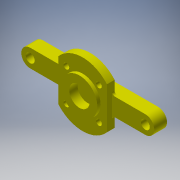
# Autodesk Inventor part: Coperchio inferiore
Saved by Autodesk Inventor 2016 (Build 200138000, 138)
## iProperties
Created: 2016-12-01
Part Number: Coperchio inferiore
Material: Generic
Document SubType Name: Modeling
Designer: Muhammad
Density: 1 g/cm^3
Appearance: Default
Author: Muhammad
Autodesk Inventor part; units mm, degrees
ref_plane "YZ Plane" through (0, 0, 0) normal (1, 0, 0) x (0, 1, 0)
ref_plane "XY Plane" through (0, 0, 0) normal (0, 0, 1) x (1, 0, 0)
sketch "Sketch1" plane through (0, 0, 0) normal (0, 1, 0) x (-1, 0, 0)
  line L0 (0, 0) -> (45, 0) construction
  line L1 (0, 0) -> (52, 0)
  line L2 (0, 0) -> (-45, 0)
  line L3 (-45, 0) -> (45, 0) construction
  line L4 (-45, -7) -> (45, -7)
  line L5 (45, 7) -> (-45, 7)
  arc A0 (-45, 7) -> (-45, -7) centre (-45, 0) ccw
  arc A1 (45, -7) -> (45, 7) centre (45, 0) ccw
  circle A2 centre (45, 0) radius 3.5
  circle A3 centre (-45, 0) radius 3.5
  dimension "d0" = 45
  dimension "d1" = 52
  dimension "d2" = 45
  dimension "d3" = 7
  constraints: 14 end point, 4 centre point, 4 point on circle, 4 tangent, 3 horizontal, 2 coincident, 1 collinear, 1 midpoint, 1 parallel
  measures "d0" distance of L0.start L0.end
  measures "d1" distance of L0.start L1.end
  measures "d2" distance of L0.start L2.end
  measures "d3" diameter of A2
extrude "Extrusion1" add sketch "Sketch1" along normal blind 10
ref_plane "Work Plane1" through (0, 2, 0) normal (0, 1, 0) x (-1, 0, 0)
sketch "Sketch2" plane through (0, 2, 0) normal (0, 1, 0) x (-1, 0, 0)
  line L0 (0, 0) -> (19, 0)
  line L1 (19, 0) -> (19, -16.2481)
  line L2 (19, 0) -> (19, 16.2481)
  line L3 (0, 0) -> (-19, 0)
  line L4 (-19, 0) -> (-19, -16.2481)
  line L5 (-19, 0) -> (-19, 16.2481)
  arc A0 (-19, -16.2481) -> (19, -16.2481) centre (0, 0) ccw
  arc A1 (19, 16.2481) -> (-19, 16.2481) centre (0, 0) ccw
  dimension "d8" = 19
  dimension "d10" = 19
  constraints: 12 end point, 4 point on circle, 2 centre point, 2 coincident, 2 horizontal, 2 point on line, 1 perpendicular, 1 vertical
  measures "d8" distance of L0.start L0.end
  measures "d10" distance of L3.start L3.end
extrude "Extrusion2" add sketch "Sketch2" against normal blind 6
fillet "Fillet1" radius 2 4 edges at (-19, 1, -7) (-19, 1, 7) (19, 1, -7) (19, 1, 7)
sketch "Sketch3" plane through (0, -4, 0) normal (0, -1, 0) x (1, 0, 0)
  circle A0 centre (0, 0) radius 18 construction
  line L0 (0, 0) -> (12.7279, 12.7279) construction
  line L1 (0, 0) -> (18, 0) construction
  circle A1 centre (12.7279, 12.7279) radius 2.25
  circle A2 centre (-12.7279, 12.7279) radius 2.25
  circle A3 centre (-12.7279, -12.7279) radius 2.25
  circle A4 centre (12.7279, -12.7279) radius 2.25
  dimension "d14" = 36
  dimension "d15" = 45
  dimension "d16" = 4.5
  dimension "d19" = 360
  constraints: 4 centre point, 4 end point, 2 coincident, 1 equal length, 1 horizontal, 12 other
  measures "d15" angle of L1 L0
  measures "d16" diameter of A1
extrude "Extrusion3" cut sketch "Sketch3" against normal blind 10
sketch "Sketch4" plane through (0, -4, 0) normal (0, -1, 0) x (1, 0, 0)
  circle A0 centre (0, 0) radius 14
  circle A1 centre (0, 0) radius 8
  dimension "d23" = 28
  dimension "d24" = 16
  constraints: 2 centre point, 2 coincident
  measures "d23" diameter of A0
  measures "d24" diameter of A1
extrude "Extrusion4" add sketch "Sketch4" along normal blind 2.5
sketch "Sketch5" plane through (0, -4, 0) normal (0, -1, 0) x (1, 0, 0)
  circle A0 centre (0, 0) radius 8
  constraints: 1 centre point, 1 coincident
extrude "Extrusion5" cut sketch "Sketch5" against normal blind 4
body "Solid1"
